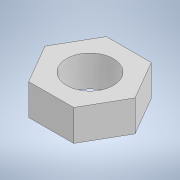
# Autodesk Inventor part: Bolt 3mm
Saved by Autodesk Inventor 2022 (Build 260153000, 153)
## iProperties
Created: 2022-06-15
Part Number: Bolt 3mm
Material: Generic
Document SubType Name: Modeling
Designer: chait
Density: 1 g/cm^3
Appearance: Default
Author: chait
Autodesk Inventor part; units mm, degrees
ref_plane "YZ Plane" through (0, 0, 0) normal (1, 0, 0) x (0, 1, 0)
ref_plane "XZ Plane" through (0, 0, 0) normal (0, 1, 0) x (-1, 0, 0)
ref_plane "XY Plane" through (0, 0, 0) normal (0, 0, 1) x (1, 0, 0)
sketch "Sketch1" plane through (0, 0, 0) normal (0, 1, 0) x (-1, 0, 0)
  line L0 (-1.4375, -2.5034) -> (-2.8867, -0.0068)
  line L1 (-2.8867, -0.0068) -> (-1.4493, 2.4966)
  line L2 (-1.4493, 2.4966) -> (1.4375, 2.5034)
  line L3 (1.4375, 2.5034) -> (2.8867, 0.0068)
  line L4 (2.8867, 0.0068) -> (1.4493, -2.4966)
  line L5 (1.4493, -2.4966) -> (-1.4375, -2.5034)
  point P0 (0, 0)
  point P1 (0, 0)
  dimension "d0" = 5
  constraints: 12 end point, 1 coincident, 13 other
  measures "d0" distance between parallel lines of L5 L2
extrude "Extrusion1" add sketch "Sketch1" along normal blind 2
sketch "Sketch3" plane through (0, 2, 0) normal (0, 1, 0) x (1, 0, 0)
  circle A0 centre (0, 0) radius 1.5
  dimension "d6" = 3
  constraints: 1 centre point, 1 coincident
  measures "d6" diameter of A0
extrude "Extrusion3" cut sketch "Sketch3" against normal blind 10
body "Solid1"
